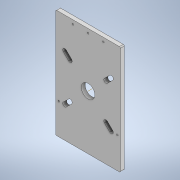
# Autodesk Inventor part: properySideGateGasket
Saved by Autodesk Inventor 2021.2 (Build 252289000, 289)
## iProperties
Created: 2020-11-21
Part Number: properySideGateGasket
Material: Generic
Document SubType Name: Modeling
Designer: robst
Density: 1 g/cm^3
Appearance: Default
Author: robst
Autodesk Inventor part; units mm, degrees
ref_plane "YZ Plane" through (0, 0, 0) normal (1, 0, 0) x (0, 1, 0)
ref_plane "XZ Plane" through (0, 0, 0) normal (0, 1, 0) x (-1, 0, 0)
ref_plane "XY Plane" through (0, 0, 0) normal (0, 0, 1) x (1, 0, 0)
sketch "Sketch2" plane through (0, 0, 0) normal (0, 0, 1) x (1, 0, 0)
  line L0 (-53, -88.9) -> (53, -88.9)
  line L1 (53, -88.9) -> (53, 88.9)
  line L2 (53, 88.9) -> (-53, 88.9)
  line L3 (-53, 88.9) -> (-53, -88.9)
  line L4 (-53, -88.9) -> (53, 88.9) construction
  line L5 (53, -88.9) -> (-53, 88.9) construction
  point P0 (0, 0)
  dimension "d0" = 106
  dimension "d1" = 177.8
  constraints: 12 end point, 2 midpoint, 2 parallel, 1 horizontal, 1 perpendicular
  measures "d0" distance of L2.end L1.end
  measures "d1" distance of L1.end L0.end
extrude "Extrusion1" add sketch "Sketch2" against normal blind 6.35
sketch "Sketch5" plane through (0, 0, 0) normal (0, 0, 1) x (1, 0, 0)
  circle A0 centre (0, 0) radius 11.1125
  dimension "d26" = 22.225
  constraints: 1 centre point, 1 coincident
  measures "d26" diameter of A0
extrude "CenterHole" cut sketch "Sketch5" against normal through all
sketch "Sketch6" plane through (0, 0, 0) normal (0, 0, 1) x (1, 0, 0)
  line L0 (-53, 88.9) -> (-53, -88.9) projected
  line L1 (53, -88.9) -> (53, 88.9) projected
  line L2 (-53, -88.9) -> (-53, 88.9) construction
  line L3 (-53, 82.4) -> (53, 82.4) construction
  line L4 (53, 88.9) -> (-53, 88.9) construction
  point P0 (0, 0)
  point P1 (0, 82.4)
  point P2 (123.3454, 23.3667)
  point P3 (-25, 82.4)
  point P4 (25, 82.4)
  dimension "d29" = 6.5
  dimension "d30" = 25
  dimension "d31" = 25
  constraints: 4 point on line, 2 end point, 1 horizontal, 1 midpoint
  measures "d29" distance between parallel lines of L3 L4
  measures "d30" distance of point (-25, 82.4) point (0, 82.4)
  measures "d31" distance of point (25, 82.4) point (0, 82.4)
hole "TopThreeHoles" at (0, 82.4, 0) at (123.3454, 23.3667, 0) at (-25, 82.4, 0) at (25, 82.4, 0) direction (0, 0, -1) diameter 2.6416 end through all thread size "6-32 UNC" class "2B" standard "ANSI Unified Screw Threads"
sketch "Sketch7" plane through (0, 0, 0) normal (0, 0, 1) x (1, 0, 0)
  line L0 (53, -88.9) -> (53, 88.9) projected
  line L1 (-53, 88.9) -> (-53, -88.9) projected
  line L2 (-53, -38.1) -> (53, -38.1) construction
  line L3 (53, 88.9) -> (53, -88.9) projected
  line L4 (53, 88.9) -> (-53, 88.9) construction
  point P0 (0, 0)
  point P1 (-48, -38.1)
  point P2 (48, -38.1)
  dimension "d39" = 127
  dimension "d40" = 5
  dimension "d41" = 5
  constraints: 4 point on line, 2 end point, 1 perpendicular
  measures "d39" distance between parallel lines of L2 L4
  measures "d40" distance from line of point (-48, -38.1) L1
  measures "d41" distance from line of point (48, -38.1) L0
hole "BottomTwoHoles" at (-48, -38.1, 0) at (48, -38.1, 0) direction (0, 0, -1) diameter 2.6416 end through all thread size "6-32 UNC" class "2B" standard "ANSI Unified Screw Threads"
fillet "Fillet1" radius 1.5875 4 edges at (53, 88.9, -3.175) (-53, 88.9, -3.175) (53, -88.9, -3.175) (-53, -88.9, -3.175)
sketch "Sketch8" plane through (0, 0, 0) normal (0, 0, 1) x (1, 0, 0)
  line L0 (0, 0) -> (-53, 53) construction
  line L1 (-53, 87.3125) -> (-53, -87.3125) construction
  line L2 (-38.0224, 38.0224) -> (-29.3295, 29.3295) construction
  line L3 (-40.4112, 35.6337) -> (-31.7183, 26.9408)
  line L4 (-26.9408, 31.7183) -> (-35.6337, 40.4112)
  arc A0 (-35.6337, 40.4112) -> (-40.4112, 35.6337) centre (-38.0224, 38.0224) ccw
  arc A1 (-31.7183, 26.9408) -> (-26.9408, 31.7183) centre (-29.3295, 29.3295) ccw
  point P0 (-33.676, 33.676)
  dimension "d50" = 45
  dimension "d51" = 6.7564
  dimension "d53" = 19.05
  dimension "d59" = 3.3782
  dimension "d60" = 41.4782
  constraints: 10 end point, 4 point on circle, 4 tangent, 3 point on line, 2 centre point, 1 midpoint, 1 parallel
  measures "d50" angle of L0 L1
  measures "d51" distance between parallel lines of L4 L3
  measures "d59" radius of A1
  measures "d60" distance of L2.end L0.start
extrude "SlotForScrews" cut sketch "Sketch8" against normal through all
pattern_circular "Circular Pattern1" count 4 over 360 about axis through (0, 0, -10) along (0, 0, 1) of "SlotForScrews"
body "Solid1"
